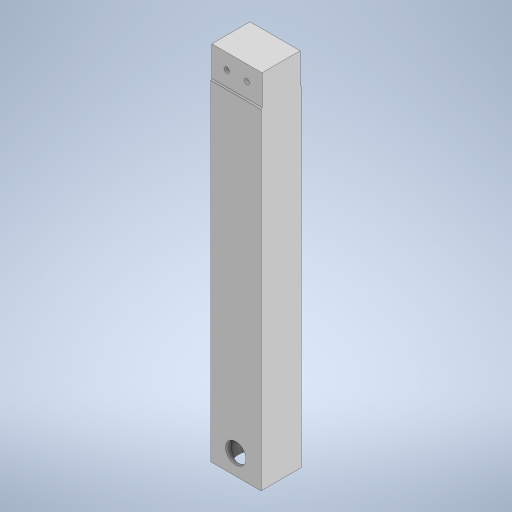
# Autodesk Inventor part: Tensile_test_bottom_adapter
Saved by Autodesk Inventor 2024 (Build 280153000, 153)
## iProperties
Created: 2023-09-15
Part Number: Tensile_test_bottom_adapter
Material: 일반
Document SubType Name: Modeling
Designer: jsw
Density: 1 g/cm^3
Appearance: 기본값
Author: jsw
Autodesk Inventor part; units mm, degrees
ref_plane "YZ Plane" through (0, 0, 0) normal (1, 0, 0) x (0, 1, 0)
ref_plane "XZ Plane" through (0, 0, 0) normal (0, 1, 0) x (-1, 0, 0)
ref_plane "XY Plane" through (0, 0, 0) normal (0, 0, 1) x (1, 0, 0)
sketch "스케치1" plane through (0, 0, 0) normal (0, 1, 0) x (-1, 0, 0)
  line L0 (-12.5, 10) -> (12.5, 10)
  line L1 (12.5, 10) -> (12.5, -10)
  line L2 (12.5, -10) -> (-12.5, -10)
  line L3 (-12.5, -10) -> (-12.5, 10)
  line L4 (-12.5, 10) -> (12.5, -10) construction
  line L5 (12.5, 10) -> (-12.5, -10) construction
  circle A0 centre (0, 0) radius 8.75
  dimension "d0" = 25
  dimension "d1" = 20
  dimension "d2" = 17.5
  constraints: 12 end point, 2 midpoint, 2 parallel, 1 centre point, 1 coincident, 1 horizontal, 1 perpendicular
  measures "d0" distance of L1.end L2.end
  measures "d1" distance of L0.end L1.end
  measures "d2" diameter of A0
extrude "돌출1" add sketch "스케치1" along normal blind 20
sketch "스케치2" plane through (12.5, 0, -10) normal (0, 0, -1) x (-1, 0, 0)
  circle A0 centre (12.5, 10) radius 5
  line L0 (0, 0) -> (25, 0) projected
  point P0 (12.5, 0)
  point P1 (12.5, 0)
  point P2 (12.5, 0)
  dimension "d5" = 10
  dimension "d6" = 10
  constraints: 2 midpoint, 1 centre point, 1 vertical alignment
  measures "d5" diameter of A0
  measures "d6" distance of point (12.5, 0) A0.centre
extrude "돌출2" cut sketch "스케치2" against normal up to surface (20 mm away)
sketch "스케치3" plane through (0, 20, 0) normal (0, 1, 0) x (1, 0, 0)
  line L0 (12.5, 10) -> (-12.5, 10) projected
  line L1 (-12.5, 10) -> (-12.5, -10) projected
  line L2 (-12.5, -10) -> (12.5, -10) projected
  line L3 (12.5, -10) -> (12.5, 10) projected
  circle A0 centre (0, 0) radius 8.75 projected
extrude "돌출3" add sketch "스케치3" along normal blind 160 contours L3 L2 L1 L0 | A0
sketch "스케치20" plane through (-12.5, 0, 10) normal (0, 0, 1) x (1, 0, 0)
  circle A0 centre (7.5, 172.5) radius 1.25
  line L0 (0, 180) -> (25, 180) projected
  line L1 (12.5, 180) -> (12.5, 173.75)
  circle A1 centre (17.5, 172.5) radius 1.25
  point P0 (12.5, 0)
  dimension "d147" = 2.5
  dimension "d151" = 7.5
  dimension "d152" = 5
  constraints: 3 midpoint, 2 centre point, 2 end point, 1 symmetric about line, 1 vertical, 1 other
  measures "d147" diameter of A0
  measures "d151" distance from line of A0.centre L0
  measures "d152" horizontal distance of A0.centre L1.start
extrude "돌출7" cut sketch "스케치20" against normal up to surface (20 mm away)
sketch "스케치21" plane through (-12.5, 0, 10) normal (0, 0, 1) x (1, 0, 0)
  line L0 (25, 180) -> (0, 180) projected
  line L1 (25, 0) -> (25, 180) projected
  line L2 (0, 180) -> (25, 180)
  line L3 (25, 180) -> (25, 165)
  line L4 (25, 165) -> (0, 165)
  line L5 (0, 165) -> (0, 180)
  point P0 (12.5, 0)
  dimension "d153" = 15
  constraints: 8 end point, 2 parallel, 1 horizontal, 1 perpendicular, 1 point on line
  measures "d153" distance of L2.end L3.end
extrude "돌출8" cut sketch "스케치21" against normal blind 0.5
ref_plane "작업 평면1" through (12.5, 0, 0) normal (0, 0, -1) x (-1, 0, 0)
mirror "미러1" about plane through (12.5, 0, 0) normal (0, 0, -1) of "돌출8"
chamfer "모따기1" distance 0.5 angle 45 2 edges at (0, 165, 10) (0, 165, -10)
equation "\"d34\" = 55deg"
equation "\"d54\" = 55deg"
equation "\"d74\" = 55deg"
equation "\"d94\" = 55deg"
equation "\"d116\" = 55deg"
equation "\"d136\" = 55deg"
